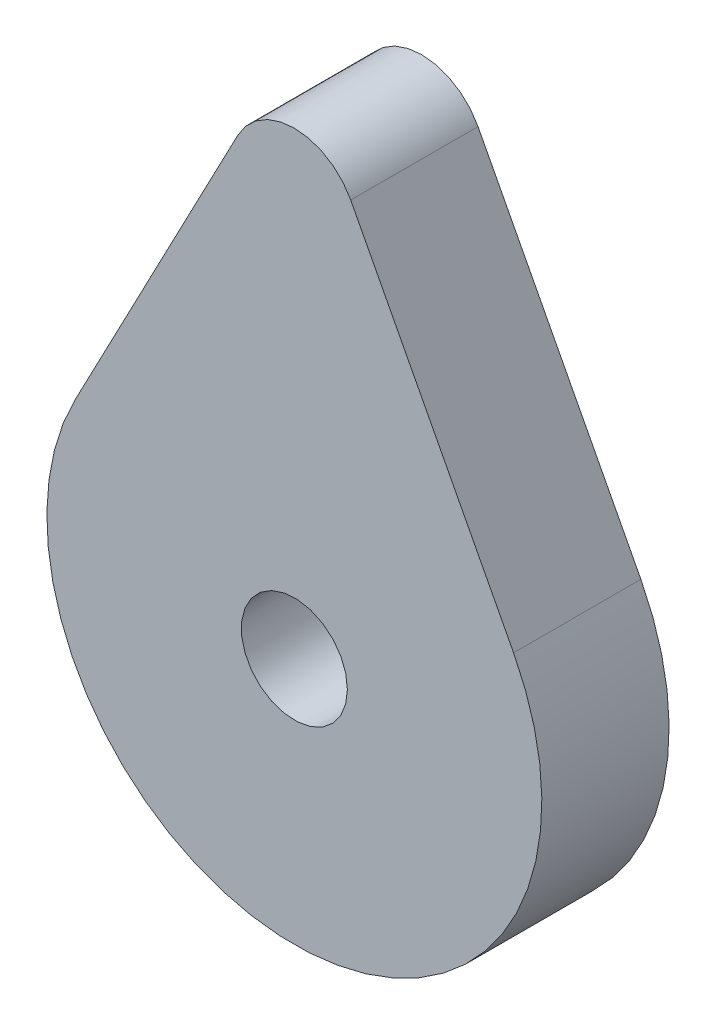
# Autodesk Inventor part: ClickSpringBacking
Saved by Autodesk Inventor 2021 (Build 250183000, 183)
## iProperties
Created: 2021-07-10
Part Number: ClickSpringBacking
Material: Generic
Document SubType Name: Modeling
Designer: teh18
Density: 1 g/cm^3
Appearance: Default
Author: teh18
Autodesk Inventor part; units mm, degrees
ref_plane "YZ Plane" through (0, 0, 0) normal (1, 0, 0) x (0, 1, 0)
ref_plane "XZ Plane" through (0, 0, 0) normal (0, 1, 0) x (-1, 0, 0)
ref_plane "XY Plane" through (0, 0, 0) normal (0, 0, 1) x (1, 0, 0)
sketch "Sketch1" plane through (0, 0, 0) normal (0, 0, 1) x (1, 0, 0)
  circle A0 centre (0, 0) radius 3.75 projected
  circle A1 centre (0, 0) radius 12.5 projected
  circle A2 centre (0, 0) radius 17.5
  line L0 (44.9276, 33.0458) -> (45.2557, 31.8342) projected
  arc A3 (45.2557, 31.8342) -> (43.9307, 28.6117) centre (50, 28) ccw projected
  line L1 (43.9307, 28.6117) -> (42.8453, 27.9812) projected
  line L2 (42.8453, 27.9812) -> (43.934, 27.3564) projected
  arc A4 (43.934, 27.3564) -> (45.2759, 24.1409) centre (50, 28) ccw projected
  line L3 (45.2759, 24.1409) -> (44.9542, 22.9276) projected
  line L4 (44.9542, 22.9276) -> (46.1658, 23.2557) projected
  arc A5 (46.1658, 23.2557) -> (49.3883, 21.9307) centre (50, 28) ccw projected
  line L5 (49.3883, 21.9307) -> (50.0188, 20.8453) projected
  line L6 (50.0188, 20.8453) -> (50.6436, 21.934) projected
  arc A6 (50.6436, 21.934) -> (53.8591, 23.2759) centre (50, 28) ccw projected
  line L7 (53.8591, 23.2759) -> (55.0724, 22.9542) projected
  line L8 (55.0724, 22.9542) -> (54.7443, 24.1658) projected
  arc A7 (54.7443, 24.1658) -> (56.0693, 27.3883) centre (50, 28) ccw projected
  line L9 (56.0693, 27.3883) -> (57.1547, 28.0188) projected
  line L10 (57.1547, 28.0188) -> (56.066, 28.6436) projected
  arc A8 (56.066, 28.6436) -> (54.7241, 31.8591) centre (50, 28) ccw projected
  line L11 (54.7241, 31.8591) -> (55.0458, 33.0724) projected
  line L12 (55.0458, 33.0724) -> (53.8342, 32.7443) projected
  arc A9 (53.8342, 32.7443) -> (50.6117, 34.0693) centre (50, 28) ccw projected
  line L13 (50.6117, 34.0693) -> (49.9812, 35.1547) projected
  line L14 (49.9812, 35.1547) -> (49.3564, 34.066) projected
  arc A10 (49.3564, 34.066) -> (46.1409, 32.7241) centre (50, 28) ccw projected
  line L15 (46.1409, 32.7241) -> (44.9276, 33.0458) projected
  circle A11 centre (50, 28) radius 20 projected
  circle A12 centre (0, 28) radius 4.5
  line L16 (15.4995, 8.125) -> (3.9856, 30.0893)
  line L17 (-3.9856, 30.0893) -> (-15.4995, 8.125)
  dimension "d0" = 35
  dimension "d3" = 9
  constraints: 4 end point, 4 point on circle, 4 tangent, 2 centre point, 1 coincident, 1 horizontal alignment, 1 vertical alignment
  measures "d0" diameter of A2
  measures "d3" diameter of A12
extrude "Extrusion1" add sketch "Sketch1" along normal blind 9 contours A1 | A2 | A2 L17 A12 L16 | A12
body "Solid1"
